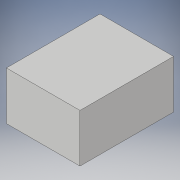
# Autodesk Inventor part: cube
Saved by Autodesk Inventor 2019 (Build 230136000, 136)
## iProperties
Created: 2021-10-28
Part Number: cube
Material: Genérico
Document SubType Name: Modeling
Designer: Juan M. Casillas
Density: 1 g/cm^3
Appearance: Valor por defecto
Author: Juan M. Casillas
Autodesk Inventor part; units mm, degrees
ref_plane "YZ Plane" through (0, 0, 0) normal (1, 0, 0) x (0, 1, 0)
ref_plane "XZ Plane" through (0, 0, 0) normal (0, 1, 0) x (-1, 0, 0)
ref_plane "XY Plane" through (0, 0, 0) normal (0, 0, 1) x (1, 0, 0)
sketch "Sketch1" plane through (0, 0, 0) normal (0, 1, 0) x (-1, 0, 0)
  line L0 (7.6348, 9.7122) -> (-7.6348, 9.7122)
  line L1 (-7.6348, 9.7122) -> (-7.6348, -9.7122)
  line L2 (-7.6348, -9.7122) -> (7.6348, -9.7122)
  line L3 (7.6348, -9.7122) -> (7.6348, 9.7122)
  line L4 (7.6348, 9.7122) -> (-7.6348, -9.7122) construction
  line L5 (-7.6348, 9.7122) -> (7.6348, -9.7122) construction
  point P0 (0, 0)
  constraints: 12 end point, 2 midpoint, 2 parallel, 1 horizontal, 1 perpendicular
extrude "Extrusion1" add sketch "Sketch1" along normal blind 10
body "Solid1"
